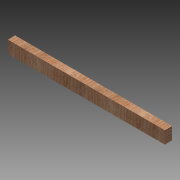
# Autodesk Inventor part: CNC-X-axis- linear drawer slider
Saved by Autodesk Inventor 2015 (Build 190159000, 159)
## iProperties
Created: 2015-03-21
Part Number: CNC-X-axis- linear drawer slider
Material: Stainless Steel
Document SubType Name: Modeling
Designer: Bangladesh
Density: 8 g/cm^3
Appearance: Semi-Polished
Author: Bangladesh
Autodesk Inventor part; units mm, degrees
ref_plane "YZ Plane" through (0, 0, 0) normal (1, 0, 0) x (0, 1, 0)
ref_plane "XZ Plane" through (0, 0, 0) normal (0, 1, 0) x (-1, 0, 0)
ref_plane "XY Plane" through (0, 0, 0) normal (0, 0, 1) x (1, 0, 0)
sketch "Sketch1" plane through (0, 0, 0) normal (0, 0, 1) x (1, 0, 0)
  line L0 (-273.05, 21.59) -> (273.05, 21.59)
  line L1 (273.05, 21.59) -> (273.05, -21.59)
  line L2 (273.05, -21.59) -> (-273.05, -21.59)
  line L3 (-273.05, -21.59) -> (-273.05, 21.59)
  line L4 (-273.05, 21.59) -> (273.05, -21.59) construction
  line L5 (273.05, 21.59) -> (-273.05, -21.59) construction
  point P0 (0, 0)
  dimension "d0" = 546.1
  dimension "d1" = 43.18
  constraints: 12 end point, 2 midpoint, 2 parallel, 1 horizontal, 1 perpendicular
  measures "d0" distance of L0.start L0.end
  measures "d1" distance of L0.end L1.end
extrude "Extrusion1" add sketch "Sketch1" along normal mid plane 25.4
body "Solid1"
